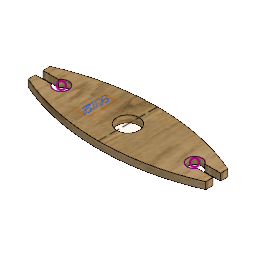
WineCaddy2Glasses v14 (Autodesk Fusion 360 design; units mm, degrees)
Autodesk Fusion 360 part; units mm, degrees
sketch "Sketch1" plane through (0, 0, 0) normal (0, 0, 1) x (1, 0, 0)
  line L0 (0, 0) -> (304.8, 0) construction
  line L1 (304.8, 0) -> (304.8, 101.6) construction
  line L2 (304.8, 101.6) -> (0, 101.6) construction
  line L3 (0, 101.6) -> (0, 0) construction
  circle A0 centre (152.4, 50.8) radius 19.05
  line L4 (0, 50.8) -> (304.8, 50.8) construction
  line L5 (27.1015, 57.15) -> (0, 57.15)
  line L6 (27.1015, 44.45) -> (0, 44.45)
  line L7 (304.8, 57.15) -> (277.6985, 57.15)
  line L8 (277.6985, 44.45) -> (304.8, 44.45)
  line L9 (0, 69.85) -> (0, 57.15)
  line L10 (0, 44.45) -> (0, 31.75)
  line L11 (304.8, 69.85) -> (304.8, 57.15)
  line L12 (304.8, 44.45) -> (304.8, 31.75)
  arc A1 (27.1015, 44.45) -> (27.1015, 57.15) centre (38.1, 50.8) ccw
  arc A2 (277.6985, 57.15) -> (277.6985, 44.45) centre (266.7, 50.8) ccw
  arc A3 (304.8, 69.85) -> (0, 69.85) centre (152.4, -280.035) ccw
  line L13 (0, 44.45) -> (304.8, 44.45) construction
  line L14 (0, 57.15) -> (304.8, 57.15) construction
  arc A4 (0, 31.75) -> (304.8, 31.75) centre (152.4, 381.635) ccw
  dimension "d1" = 304.8
  dimension "d2" = 101.6
  dimension "d3" = 38.1
  dimension "d5" = 152.4
  dimension "d6" = 25.4
  dimension "d7" = 25.4
  dimension "d8" = 38.1
  dimension "d9" = 38.1
  dimension "d12" = 6.35
  dimension "d13" = 6.35
  dimension "d14" = 12.7
  dimension "d18" = 12.7
  measures "d3" diameter of A0
  measures "d6" diameter of A1
  measures "d7" diameter of A2
extrude "Extrude1" add sketch "Sketch1" along normal blind 12.1412
sketch "Sketch2" plane through (0, 0, 12.1412) normal (0, 0, 1) x (-1, 0, 0)
  circle A0 centre (-152.4, -50.8) radius 19.05
  line L0 (-277.6985, -57.15) -> (-304.8, -57.15)
  line L1 (-304.8, -57.15) -> (-304.8, -69.85)
  arc A1 (-304.8, -69.85) -> (0, -69.85) centre (-152.4, 280.035) ccw
  line L2 (0, -69.85) -> (0, -57.15)
  line L3 (0, -57.15) -> (-27.1015, -57.15)
  line L4 (-27.1015, -44.45) -> (0, -44.45)
  line L5 (0, -44.45) -> (0, -31.75)
  arc A2 (0, -31.75) -> (-304.8, -31.75) centre (-152.4, -381.635) ccw
  line L6 (-304.8, -31.75) -> (-304.8, -44.45)
  line L7 (-304.8, -44.45) -> (-277.6985, -44.45)
  line L8 (-89.0222, -74.9883) -> (-89.0222, -26.3401) construction
  line L9 (-89.0222, -26.3401) -> (-108.0722, -26.3401) construction
  line L10 (-108.0722, -26.3401) -> (-108.0722, -74.9883) construction
  line L11 (-108.0722, -74.9883) -> (-89.0222, -74.9883) construction
  line L12 (-152.4, -101.6) -> (-152.4, 0) construction
  arc A3 (-277.6985, -57.15) -> (-277.6985, -44.45) centre (-266.7, -50.8) ccw
  arc A4 (-27.1015, -44.45) -> (-27.1015, -57.15) centre (-38.1, -50.8) ccw
